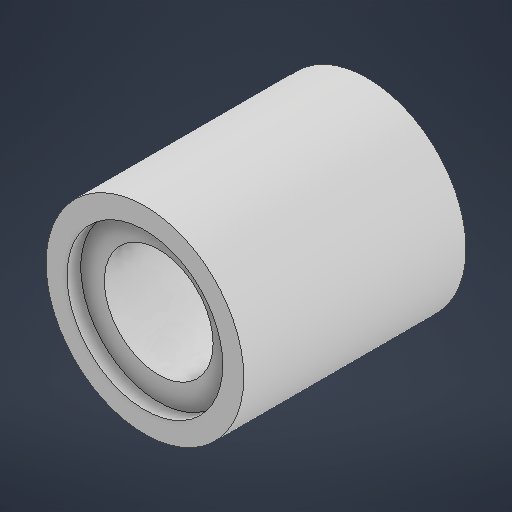
# Autodesk Inventor part: CH3-DiffBoxSpacers
Saved by Autodesk Inventor 2026.1 (Build 301233020, 233B)
## iProperties
Created: 2025-10-22
Part Number: CH3-DiffBoxSpacers
Material: Generic
Document SubType Name: Modeling
Designer: johnh
Density: 1 g/cm^3
Appearance: Default
Author: johnh
Autodesk Inventor part; units mm, degrees
ref_plane "YZ Plane" through (0, 0, 0) normal (1, 0, 0) x (0, 1, 0)
ref_plane "XZ Plane" through (0, 0, 0) normal (0, 1, 0) x (-1, 0, 0)
ref_plane "XY Plane" through (0, 0, 0) normal (0, 0, 1) x (1, 0, 0)
sketch "Sketch1" plane through (0, 0, 0) normal (0, 0, 1) x (1, 0, 0)
  circle A0 centre (0, 0) radius 6.985
  circle A1 centre (0, 0) radius 12.7
  circle A2 centre (0, 0) radius 10.0076
  dimension "d0" = 25.4
  dimension "d1" = 13.97
  dimension "d4" = 20.0152
  constraints: 3 centre point, 3 coincident
  measures "d0" diameter of A1
  measures "d1" diameter of A0
  measures "d4" diameter of A2
extrude "Extrusion1" add sketch "Sketch1" against normal blind 28.5496 contours A1 | A2
extrude "Extrusion2" cut sketch "Sketch1" against normal blind 1.778 contours A2
body "Solid1"
